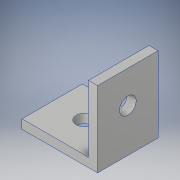
# Autodesk Inventor part: Mounting Bracket 2
Saved by Autodesk Inventor 2019.4 (Build 234330000, 330)
## iProperties
Created: 2020-01-24
Part Number: Mounting Bracket 2
Material: Aluminum 6061
Document SubType Name: Modeling
Designer: admin
Density: 2.7 g/cm^3
Appearance: Aluminum - Flat
Author: admin
Autodesk Inventor part; units mm, degrees
ref_plane "YZ Plane" through (0, 0, 0) normal (1, 0, 0) x (0, 1, 0)
ref_plane "XZ Plane" through (0, 0, 0) normal (0, 1, 0) x (-1, 0, 0)
sketch "Sketch1" plane through (0, 0, 0) normal (0, 0, 1) x (1, 0, 0)
  line L0 (0, 0) -> (0, 25)
  line L1 (0, 25) -> (-3, 25)
  line L2 (-3, 25) -> (-3, 3)
  line L3 (-3, 3) -> (-25, 3)
  line L4 (-25, 3) -> (-25, 0)
  line L5 (-25, 0) -> (0, 0)
  dimension "d0" = 3
  dimension "d1" = 3
  dimension "d2" = 25
  dimension "d3" = 25
  constraints: 12 end point, 4 perpendicular, 2 vertical
  measures "d0" distance between parallel lines of L5 L3
  measures "d1" distance between parallel lines of L0 L2
  measures "d2" distance of L4.end L0.start
  measures "d3" distance of L0.start L0.end
extrude "Extrusion1" add sketch "Sketch1" along normal blind 20
sketch "Sketch2" plane through (-25, 3, 0) normal (0, 1, 0) x (1, 0, 0)
  circle A0 centre (10.7, -10) radius 2.75
  line L0 (25, 0) -> (25, -20) projected
  line L1 (22, 0) -> (0, 0) projected
  dimension "d6" = 5.5
  dimension "d7" = 14.3
  dimension "d8" = 10
  constraints: 1 centre point
  measures "d6" diameter of A0
  measures "d7" distance from line of L0 A0.centre
  measures "d8" distance from line of L1 A0.centre
extrude "Extrusion2" cut sketch "Sketch2" against normal through all
ref_plane "Work Plane1" through (-3, 3, 0) normal (0.7071, 0.7071, 0) x (0, 0, 1)
mirror "Mirror1" about plane through (-3, 3, 0) normal (0.7071, 0.7071, 0) of "Extrusion2"
body "Solid1"
